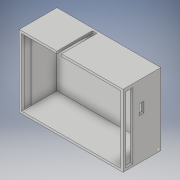
# Autodesk Inventor part: case-v3
Saved by Autodesk Inventor 2018.3 (Build 223284000, 284)
## iProperties
Created: 2019-04-23
Part Number: case-v3
Material: Generic
Document SubType Name: Modeling
Designer: Carlos Lopez
Density: 1 g/cm^3
Appearance: Default
Author: Carlos Lopez
Autodesk Inventor part; units mm, degrees
ref_plane "YZ Plane" through (0, 0, 0) normal (1, 0, 0) x (0, 1, 0)
ref_plane "XZ Plane" through (0, 0, 0) normal (0, 1, 0) x (-1, 0, 0)
ref_plane "XY Plane" through (0, 0, 0) normal (0, 0, 1) x (1, 0, 0)
sketch "Sketch1" plane through (0, 0, 0) normal (0, 0, 1) x (1, 0, 0)
  line L0 (0, 0) -> (83.9978, 0)
  line L1 (83.9978, 0) -> (83.9978, 56.9999)
  line L2 (83.9978, 56.9999) -> (0, 56.9999)
  line L3 (0, 56.9999) -> (0, 0)
  dimension "d0" = 83.9978
  dimension "d1" = 56.9999
  constraints: 8 end point, 2 parallel, 1 horizontal, 1 perpendicular
  measures "d0" distance of L2.end L1.end
  measures "d1" distance of L1.end L0.end
extrude "Extrusion1" add sketch "Sketch1" along normal blind 29.9999
shell "Shell1" thickness 2 outward yes removed faces 1 at (27.9993, 37.9999, 29.9999)
sketch "Sketch2" plane through (85.9978, -2, -2) normal (1, 0, 0) x (0, 0, -1)
  point P0 (-2, 2)
sketch "Sketch3" plane through (85.9978, -2, -2) normal (1, 0, 0) x (0, 0, -1)
  line L0 (-2, 58.9999) -> (-31.9999, 58.9999) projected
  line L1 (-29.6685, 58.1425) -> (-23.6741, 58.1425)
  line L2 (-23.6741, 58.1425) -> (-23.6741, 2.1426)
  line L3 (-23.6741, 2.1426) -> (-29.6685, 2.1426)
  line L4 (-29.6685, 2.1426) -> (-29.6685, 58.1425)
  point P0 (-2, 2)
  dimension "d5" = 5.9944
  dimension "d6" = 55.9999
  constraints: 8 end point, 2 parallel, 1 horizontal, 1 perpendicular
  measures "d5" distance of L2.end L3.end
  measures "d6" distance of L1.end L2.end
extrude "Extrusion2" cut sketch "Sketch3" against normal blind 87.0001
sketch "Sketch4" plane through (85.9978, -2, -2) normal (1, 0, 0) x (0, 0, -1)
  line L0 (-14.3813, 35.0012) -> (-18.3691, 35.0012)
  line L1 (-18.3691, 35.0012) -> (-18.3691, 43.5102)
  line L2 (-18.3691, 43.5102) -> (-14.3813, 43.5102)
  line L3 (-14.3813, 43.5102) -> (-14.3813, 35.0012)
  point P0 (-2, 2)
  point P1 (-13.7922, 50.8)
  dimension "d9" = 3.9878
  dimension "d10" = 8.509
  constraints: 8 end point, 2 parallel, 1 horizontal, 1 perpendicular
  measures "d9" distance of L1.end L2.end
  measures "d10" distance of L0.end L1.end
extrude "Extrusion3" cut sketch "Sketch4" against normal blind 12.7
sketch "Sketch5" plane through (-2, 58.9999, -2) normal (0, 1, 0) x (1, 0, 0)
  line L0 (85.9978, -31.9999) -> (2, -31.9999) projected
  line L1 (31.9983, -31.9999) -> (35.9099, -31.9999)
  line L2 (35.9099, -31.9999) -> (35.9099, -2)
  line L3 (35.9099, -2) -> (31.9983, -2)
  line L4 (31.9983, -2) -> (31.9983, -31.9999)
  point P0 (2, -2)
  dimension "d13" = 3.9116
  constraints: 8 end point, 2 parallel, 1 horizontal, 1 perpendicular, 1 point on line
  measures "d13" distance of L3.end L2.end
extrude "Extrusion4" cut sketch "Sketch5" against normal blind 12.7
body "Solid1"
